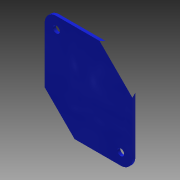
# Autodesk Inventor part: plaat
Saved by Autodesk Inventor 2015 (Build 190159000, 159)
## iProperties
Created: 2016-01-19
Part Number: plaat
Material: Generic
Document SubType Name: Modeling
Designer: david
Density: 1 g/cm^3
Appearance: Blue - Wall Paint - Glossy
Author: david
Autodesk Inventor part; units mm, degrees
ref_plane "YZ Plane" through (0, 0, 0) normal (1, 0, 0) x (0, 1, 0)
ref_plane "XZ Plane" through (0, 0, 0) normal (0, 1, 0) x (-1, 0, 0)
ref_plane "XY Plane" through (0, 0, 0) normal (0, 0, 1) x (1, 0, 0)
sketch "Sketch1" plane through (0, 0, 0) normal (0, 1, 0) x (-1, 0, 0)
  line L0 (-16.5, 25) -> (16.5, 25)
  line L1 (22.5, 19) -> (22.5, -19)
  line L2 (16.5, -25) -> (-16.5, -25)
  line L3 (-22.5, -19) -> (-22.5, 19)
  line L4 (-22.5, 25) -> (22.5, -25) construction
  line L5 (22.5, 25) -> (-22.5, -25) construction
  arc A0 (16.5, -25) -> (22.5, -19) centre (16.5, -19) ccw
  arc A1 (22.5, 19) -> (16.5, 25) centre (16.5, 19) ccw
  arc A2 (-16.5, 25) -> (-22.5, 19) centre (-16.5, 19) ccw
  arc A3 (-22.5, -19) -> (-16.5, -25) centre (-16.5, -19) ccw
  point P0 (0, 0)
  dimension "d0" = 45
  dimension "d1" = 50
  dimension "d2" = 6
  constraints: 12 end point, 8 point on circle, 8 point on line, 8 tangent, 4 centre point, 3 equal radius, 2 midpoint, 2 parallel, 1 horizontal, 1 perpendicular
  measures "d0" distance of L4.end L5.end
  measures "d1" distance of L5.start L4.end
  measures "d2" radius of A0
extrude "Extrusion1" add sketch "Sketch1" along normal blind 1.5
sketch "Sketch2" plane through (0, 1.5, 0) normal (0, 1, 0) x (1, 0, 0)
  arc A0 (-22.5, -19) -> (-16.5, -25) centre (-16.5, -19) ccw projected
  circle A1 centre (-16.5, -19) radius 1.75
  arc A2 (-16.5, 25) -> (-22.5, 19) centre (-16.5, 19) ccw projected
  circle A3 centre (-16.5, 19) radius 1.75
  arc A4 (22.5, 19) -> (16.5, 25) centre (16.5, 19) ccw projected
  circle A5 centre (16.5, 19) radius 1.75
  arc A6 (16.5, -25) -> (22.5, -19) centre (16.5, -19) ccw projected
  circle A7 centre (16.5, -19) radius 1.75
  point P0 (0, 0)
  dimension "d5" = 3.5
  dimension "d6" = 3.5
  dimension "d7" = 3.5
  dimension "d8" = 3.5
  constraints: 4 centre point, 4 coincident
  measures "d5" diameter of A1
  measures "d6" diameter of A3
  measures "d7" diameter of A5
  measures "d8" diameter of A7
extrude "Extrusion2" cut sketch "Sketch2" against normal blind 1.5
body "Solid1"
